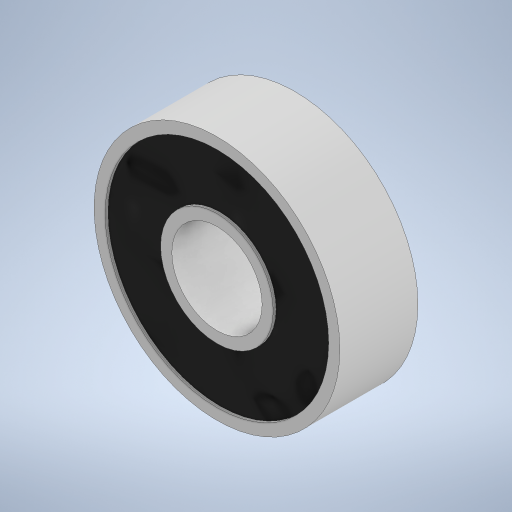
# Autodesk Inventor part: bearing_22x8x7
Saved by Autodesk Inventor 2023 (Build 270158000, 158)
## iProperties
Created: 2023-11-23
Part Number: bearing_22x8x7
Material: Generic
Document SubType Name: Modeling
Designer: aaron
Density: 1 g/cm^3
Appearance: Default
Author: aaron
Autodesk Inventor part; units mm, degrees
ref_plane "YZ Plane" through (0, 0, 0) normal (1, 0, 0) x (0, 1, 0)
ref_plane "XZ Plane" through (0, 0, 0) normal (0, 1, 0) x (-1, 0, 0)
ref_plane "XY Plane" through (0, 0, 0) normal (0, 0, 1) x (1, 0, 0)
sketch "Sketch1" plane through (0, 0, 0) normal (0, 0, 1) x (1, 0, 0)
  circle A0 centre (0, 0) radius 11.025
  circle A1 centre (0, 0) radius 4.05
  dimension "d0" = 22.05
  dimension "d1" = 8.1
  constraints: 2 centre point, 2 coincident
  measures "d0" diameter of A0
  measures "d1" diameter of A1
extrude "Extrusion1" add sketch "Sketch1" along normal blind 7
sketch "Sketch2" plane through (0, 0, 7) normal (0, 0, 1) x (1, 0, 0)
  circle A0 centre (0, 0) radius 5.05
  circle A1 centre (0, 0) radius 10.025
  circle A2 centre (0, 0) radius 11.025 projected
  circle A3 centre (0, 0) radius 4.05 projected
  dimension "d4" = 1
  dimension "d5" = 1
  constraints: 2 centre point, 2 coincident
  measures "d4" radial gap between concentric circles of A1 A2
  measures "d5" radial gap between concentric circles of A3 A0
extrude "Extrusion2" cut sketch "Sketch2" against normal blind 0.25 contours A1
sketch "Sketch3" plane through (0, 0, 0) normal (0, 0, -1) x (-1, 0, 0)
  circle A0 centre (0, 0) radius 10.025 projected
  circle A1 centre (0, 0) radius 5.05 projected
extrude "Extrusion3" cut sketch "Sketch3" against normal blind 0.25
body "Solid1"
